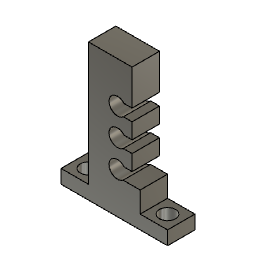
Horizantal Holder design v7 (Autodesk Fusion 360 archive; units mm, degrees)
design "Single Julia design"
Autodesk Fusion 360 part; units mm, degrees
box "BoxPrimitive2" add length 25.4 width 76.2 height 2.54 placed x (0, 0, 1) y (1, 0, 0) z (0, 1, 0) at (0, 0, 0)
sketch "Sketch3" plane through (0, 2.54, 0) normal (0, 1, 0) x (-1, 0, 0)
  line L0 (0, 25.4) -> (-76.2, 25.4)
  line L1 (-76.2, 0) -> (0, 0)
  line L2 (0, 0) -> (0, 25.4)
  line L3 (-29.21, 12.7) -> (-19.05, 12.7)
  line L4 (-19.05, 12.7) -> (-19.05, 25.4)
  line L5 (-19.05, 25.4) -> (-15.875, 25.4)
  line L6 (-15.875, 25.4) -> (-15.875, 0)
  line L7 (-15.875, 0) -> (-19.05, 0)
  line L8 (-19.05, 0) -> (-19.05, 12.7)
  line L9 (-15.875, 12.7) -> (-12.065, 12.7)
  line L10 (-12.065, 12.7) -> (-12.065, 25.4)
  line L11 (-12.065, 12.7) -> (-12.065, 0)
  line L12 (-17.4625, 25.4) -> (-17.4625, 0)
  circle A0 centre (-17.4625, 12.7) radius 1.5875
  circle A1 centre (-17.4625, 17.78) radius 1.5875
  circle A2 centre (-17.4625, 7.62) radius 1.5875
  line L13 (-19.05, 0) -> (-24.13, 0)
  line L14 (-24.13, 0) -> (-24.13, 2.54)
  line L15 (-24.13, 2.54) -> (-19.05, 2.54)
  line L16 (-19.05, 2.54) -> (-19.05, 0)
  line L17 (-19.05, 0) -> (-24.13, 0)
  line L18 (-24.13, 0) -> (-24.13, 2.54)
  dimension "d29" = 10.16
  dimension "d30" = 3.175
  dimension "d31" = 3.175
  dimension "d32" = 3.81
  dimension "d51" = 3.175
  dimension "d52" = 3.175
  dimension "d53" = 3.175
  dimension "d80" = 5.08
  dimension "d81" = 2.54
  constraint perpendicular L3 L4
  constraint perpendicular L4 L5
  constraint coincident L1 L6.end
  constraint perpendicular L1 L6
  constraint perpendicular L6 L7
  constraint midpoint L6 L9.start
  constraint perpendicular L6 L9
  constraint coincident L0 L10.end
  constraint perpendicular L0 L10
  constraint coincident L1 L11.end
  constraint perpendicular L1 L11
  constraint midpoint L5 L12.start
  constraint midpoint L7 L12.end
  constraint midpoint L12 A0.centre
  constraint coincident L12 A1.centre
  constraint coincident L12 A2.centre
  constraint perpendicular L8 L13
  constraint perpendicular L1 L14
  constraint horizontal L15
  constraint vertical L16
  constraint horizontal L17
  constraint vertical L18
  measures "d29" distance of L3.start L3.end
  measures "d30" distance of L4.end L5.end
  measures "d31" distance of L6.end L7.end
  measures "d32" distance of L9.start L9.end
  measures "d51" diameter of A0
  measures "d52" diameter of A1
  measures "d53" diameter of A2
  measures "d80" distance of L7.end L13.end
  measures "d81" distance of L13.end L14.end
scale "Scale1" factors (0.841667, 1, 1) about (0, 2.54, 25.4) bodies 1
move_body "Move1" bodies 1 to x (1, 0, 0) y (0, 1, 0) z (0, 0, 1) at (12.065, 0, 0)
extrude "Extrude1" cut sketch "Sketch3" against normal blind 12.7 contours L12 A1 | L12 A0 | L12 A1 | L12 A2 | L12 A0 | L12 A2
sketch "Sketch4" plane through (76.2, 0, 0) normal (1, 0, 0) x (0, 1, 0)
  line L0 (2.54, 25.4) -> (0, 25.4)
  line L1 (0, 25.4) -> (0, 0)
  line L2 (0, 0) -> (2.54, 0)
  line L3 (2.54, 0) -> (2.54, 25.4)
  line L4 (2.54, 0) -> (2.54, 2.54)
  line L5 (0, 2.54) -> (2.54, 2.54)
  line L6 (0, 2.54) -> (0, 0)
  line L7 (2.54, 0) -> (0, 0)
  dimension "d56" = 2.54
  constraint coincident L2.end L3.start
  constraint coincident L3 L4.end
  constraint coincident L1 L5.start
  constraint perpendicular L4 L5
  constraint coincident L1.end L2.start
  measures "d56" distance of L2.end L4.end
extrude "Extrude2" add sketch "Sketch4" along normal blind 5.08 contours L1 L2 L3 L4 L5 L6 L7
sketch "Sketch5" plane through (12.065, 0, 0) normal (-1, 0, 0) x (0, -1, 0)
  line L0 (-2.54, 0) -> (0, 0)
  line L1 (0, 0) -> (0, 25.4)
  line L2 (0, 25.4) -> (-2.54, 25.4)
  line L3 (-2.54, 25.4) -> (-2.54, 0)
  line L4 (0, 0) -> (0, 2.54)
  line L5 (0, 2.54) -> (-2.54, 2.54)
  line L6 (-2.54, 0) -> (-2.54, 2.54)
  line L7 (-2.54, 0) -> (0, 0)
  dimension "d59" = 2.54
  constraint coincident L0.end L1.start
  constraint perpendicular L0 L4
  constraint coincident L3 L5.end
  constraint perpendicular L3 L5
  constraint coincident L0.start L3.end
  measures "d59" distance of L0.end L4.end
extrude "Extrude3" add sketch "Sketch5" along normal blind 5.08 contours L0 L1 L3 L4 L5 L6 L7
move_face "MoveFace1" by (0, 2.54, 0) 1 faces at (57.15, 2.54, 13.5467)
sketch "Sketch7" plane through (0, 0, 2.54) normal (0, 0, 1) x (-1, 0, 0)
  line L0 (-76.2, -5.08) -> (-76.2, 0)
  line L1 (-76.2, 0) -> (-81.28, 0)
  line L2 (-81.28, 0) -> (-81.28, -5.08)
  line L3 (-81.28, -5.08) -> (-76.2, -5.08)
  line L4 (-81.28, -5.08) -> (-81.28, -2.54)
  line L5 (-78.74, -2.54) -> (-78.74, -5.08)
  circle A0 centre (-78.74, -2.54) radius 1.5
  dimension "d63" = 3
  constraint coincident L2.end L3.start
  constraint midpoint L2 L4.end
  constraint midpoint L3 L5.end
  constraint perpendicular L3 L5
  constraint coincident L5.start A0.centre
  measures "d63" diameter of A0
sketch "Sketch8" plane through (0, 0, 2.54) normal (0, 0, 1) x (-1, 0, 0)
  line L0 (-12.065, 0) -> (-12.065, -5.08)
  line L1 (-12.065, -5.08) -> (-6.985, -5.08)
  line L2 (-6.985, -5.08) -> (-6.985, 0)
  line L3 (-6.985, 0) -> (-12.065, 0)
  line L4 (-6.985, -2.54) -> (-9.525, -2.54)
  circle A0 centre (-9.525, -2.54) radius 1.5
  dimension "d64" = 3
  constraint midpoint L2 L4.start
  constraint perpendicular L2 L4
  constraint coincident L4.end A0.centre
  measures "d64" diameter of A0
extrude "Extrude4" cut sketch "Sketch8" sketch "Sketch7" against normal blind 5 contours A0 of sketch 2 contours A0
sketch "Sketch9" plane through (0, 0, 0) normal (0, 1, 0) x (1, 0, 0)
  line L0 (18.6768, -18.816) -> (20.1542, -18.816)
  line L1 (20.1542, -18.816) -> (20.1542, -26.2967)
  line L2 (20.1542, -26.2967) -> (21.6542, -26.2967)
  line L3 (21.6542, -26.2967) -> (21.6542, -16.6091)
  line L4 (18.1034, -16.6091) -> (18.1034, -18.816)
  line L5 (18.1034, -18.816) -> (18.6768, -18.816)
  line L6 (18.1034, -11.5091) -> (18.1034, -13.716)
  line L7 (18.1034, -13.716) -> (18.6768, -13.716)
  line L8 (18.6768, -13.716) -> (20.1542, -13.716)
  line L9 (20.1542, -13.716) -> (20.1542, -16.6091)
  line L10 (20.1542, -16.6091) -> (18.1034, -16.6091)
  line L11 (18.1034, -8.616) -> (18.6768, -8.616)
  line L12 (18.6768, -8.616) -> (20.1542, -8.616)
  line L13 (21.6542, -6.4091) -> (18.1034, -6.4091)
  line L14 (18.1034, -6.4091) -> (18.1034, -8.616)
  line L15 (21.6542, -6.4091) -> (21.6542, -16.6091)
  line L16 (20.1542, -8.616) -> (20.1542, -11.5091)
  line L17 (20.1542, -11.5091) -> (18.1034, -11.5091)
  dimension "d67" = 1.5
  constraint horizontal L0
  constraint perpendicular L0 L1
  constraint perpendicular L1 L2
  constraint perpendicular L2 L3
  constraint perpendicular L0 L4
  constraint perpendicular L4 L5
  constraint horizontal L8
  constraint perpendicular L6 L8
  constraint perpendicular L6 L7
  constraint perpendicular L8 L9
  constraint perpendicular L4 L10
  constraint horizontal L12
  constraint perpendicular L12 L14
  constraint perpendicular L11 L14
  constraint perpendicular L13 L15
  constraint perpendicular L12 L16
  constraint perpendicular L6 L17
  measures "d67" distance of L1.end L2.end
extrude "Extrude5" cut sketch "Sketch9" along normal blind 11
sketch "Sketch10" plane through (0, 0, 0) normal (0, -1, 0) x (1, 0, 0)
  line L0 (18.6823, 13.716) -> (20.1542, 13.716)
  line L1 (20.1542, 13.716) -> (20.1542, 16.6091)
  line L2 (20.1542, 16.6091) -> (18.5345, 16.6091)
  arc A0 (18.6654, 18.816) -> (18.5345, 16.6091) centre (17.4625, 17.78) ccw
  line L3 (18.6654, 18.816) -> (20.1542, 18.816)
  line L4 (20.1542, 18.816) -> (20.1542, 25.4)
  line L5 (20.1542, 25.4) -> (12.065, 25.4)
  line L6 (12.065, 25.4) -> (12.065, 2.54)
  line L7 (12.065, 2.54) -> (6.985, 2.54)
  line L8 (6.985, 2.54) -> (6.985, 0)
  line L9 (6.985, 0) -> (81.28, 0)
  line L10 (81.28, 0) -> (81.28, 2.54)
  line L11 (81.28, 2.54) -> (76.2, 2.54)
  line L12 (76.2, 2.54) -> (76.2, 25.4)
  line L13 (76.2, 25.4) -> (21.6542, 25.4)
  line L14 (21.6542, 25.4) -> (21.6542, 6.4091)
  line L15 (21.6542, 6.4091) -> (18.4891, 6.4091)
  arc A1 (18.6987, 8.616) -> (18.4891, 6.4091) centre (17.4625, 7.62) ccw
  line L16 (18.6987, 8.616) -> (20.1542, 8.616)
  line L17 (20.1542, 8.616) -> (20.1542, 11.5091)
  line L18 (20.1542, 11.5091) -> (18.5122, 11.5091)
  arc A2 (18.6823, 13.716) -> (18.5122, 11.5091) centre (17.4625, 12.7) ccw
  line L19 (21.6542, 25.4) -> (81.28, 25.4)
  line L20 (81.28, 25.4) -> (81.28, 0)
  line L21 (81.28, 0) -> (21.6542, 0)
  line L22 (21.6542, 0) -> (21.6542, 25.4)
  constraint horizontal L19
  constraint vertical L20
  constraint horizontal L21
  constraint vertical L22
  constraint coincident L9.end L10.start
  constraint coincident L13.end L14.start
extrude "Extrude6" cut sketch "Sketch10" against normal blind 7 contours L9 L10 L11 L12 L13 L14 L19 L20 L21 L22
sketch "Sketch11" plane through (0, 0, 0) normal (0, -1, 0) x (1, 0, 0)
  line L0 (21.6542, 0) -> (21.6542, 6.4091)
  line L1 (21.6542, 6.4091) -> (18.4891, 6.4091)
  arc A0 (18.6987, 8.616) -> (18.4891, 6.4091) centre (17.4625, 7.62) ccw
  line L2 (18.6987, 8.616) -> (20.1542, 8.616)
  line L3 (20.1542, 8.616) -> (20.1542, 11.5091)
  line L4 (20.1542, 11.5091) -> (18.5122, 11.5091)
  arc A1 (18.6823, 13.716) -> (18.5122, 11.5091) centre (17.4625, 12.7) ccw
  line L5 (18.6823, 13.716) -> (20.1542, 13.716)
  line L6 (20.1542, 13.716) -> (20.1542, 16.6091)
  line L7 (20.1542, 16.6091) -> (18.5345, 16.6091)
  arc A2 (18.6654, 18.816) -> (18.5345, 16.6091) centre (17.4625, 17.78) ccw
  line L8 (18.6654, 18.816) -> (20.1542, 18.816)
  line L9 (20.1542, 18.816) -> (20.1542, 25.4)
  line L10 (20.1542, 25.4) -> (12.065, 25.4)
  line L11 (12.065, 25.4) -> (12.065, 2.54)
  line L12 (12.065, 2.54) -> (6.985, 2.54)
  line L13 (6.985, 2.54) -> (6.985, 0)
  line L14 (6.985, 0) -> (21.6542, 0)
  line L15 (6.985, 2.54) -> (30, 2.54)
  line L16 (21.6542, 2.54) -> (26.7342, 2.54)
  line L17 (26.7342, 2.54) -> (26.7342, 0)
  line L18 (26.7342, 0) -> (21.6542, 0)
  line L19 (21.6542, 0) -> (21.6542, 2.54)
  dimension "d84" = 5.08
  constraint coincident L12.end L13.start
  constraint perpendicular L0 L15
  constraint horizontal L16
  constraint vertical L17
  constraint horizontal L18
  constraint vertical L19
  constraint coincident L15 L16.start
  constraint coincident L0 L16.start
  measures "d84" distance of L16.start L16.end
extrude "Extrude7" add sketch "Sketch11" against normal blind 5.08 contours L0 L15 L16 L17 L18 L19
sketch "Sketch12" plane through (0, 0, 2.54) normal (0, 0, 1) x (-1, 0, 0)
  line L0 (-21.6542, 0) -> (-26.7342, 0)
  line L1 (-26.7342, 0) -> (-26.7342, -5.08)
  line L2 (-26.7342, -5.08) -> (-21.6542, -5.08)
  line L3 (-21.6542, -5.08) -> (-21.6542, 0)
  line L4 (-26.7342, -2.54) -> (-24.1942, -2.54)
  circle A0 centre (-24.1942, -2.54) radius 1.5
  dimension "d87" = 2.54
  dimension "d88" = 3
  constraint midpoint L1 L4.start
  constraint perpendicular L1 L4
  constraint coincident L4.end A0.centre
  measures "d87" distance of L4.start L4.end
  measures "d88" diameter of A0
extrude "Extrude8" cut sketch "Sketch12" against normal blind 4 contours A0
sketch "Sketch13" plane through (0, 0, 0) normal (0, 0, -1) x (1, 0, 0)
  circle A0 centre (24.1942, -2.54) radius 1.5
  line L0 (26.7342, 0) -> (6.985, 0)
  line L1 (6.985, 0) -> (6.985, -5.08)
  line L2 (6.985, -5.08) -> (26.7342, -5.08)
  line L3 (26.7342, -5.08) -> (26.7342, 0)
  circle A1 centre (9.525, -2.54) radius 1.5

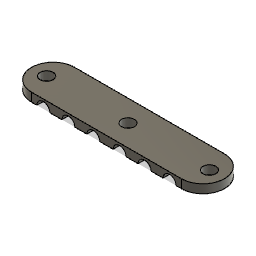
design "ESc indie mount"
Autodesk Fusion 360 part; units mm, degrees
sketch "Sketch1" plane through (0, 0, 0) normal (0, 0, 1) x (1, 0, 0)
  line L0 (0, 0) -> (17.1, 0)
  line L1 (17.1, 0) -> (17.1, 2)
  line L2 (17.1, 2) -> (0, 2)
  line L3 (0, 2) -> (0, 0)
  line L4 (0, 0) -> (1.25, 0)
  line L5 (1.25, 0) -> (2.75, 0)
  circle A0 centre (2.75, 0) radius 1.5
  line L6 (4.25, 0) -> (7.05, 0)
  line L7 (7.05, 0) -> (8.55, 0)
  circle A1 centre (8.55, 0) radius 1.5
  line L8 (10.05, 0) -> (12.85, 0)
  line L9 (12.85, 0) -> (14.35, 0)
  circle A2 centre (14.35, 0) radius 1.5
  line L10 (15.85, 0) -> (17.1, 0)
  line L11 (15.85, 0) -> (17.4, 0)
  line L12 (17.4, 0) -> (18.95, 0)
  line L13 (18.95, 0) -> (17.1, 0)
  line L14 (17.1, 0) -> (17.1, 2)
  line L15 (17.1, 2) -> (18.95, 2)
  line L16 (18.95, 2) -> (18.95, 0)
  line L17 (17.1, 2) -> (34.2, 2)
  line L18 (34.2, 0) -> (17.1, 0)
  line L19 (18.95, 0) -> (20.45, 0)
  circle A3 centre (20.45, 0) radius 1.5
  line L20 (21.95, 0) -> (24.75, 0)
  line L21 (24.75, 0) -> (26.25, 0)
  circle A4 centre (26.25, 0) radius 1.5
  line L22 (27.75, 0) -> (30.55, 0)
  line L23 (30.55, 0) -> (32.05, 0)
  circle A5 centre (32.05, 0) radius 1.5
  line L24 (33.55, 0) -> (34.8, 0)
  line L25 (34.8, 0) -> (33.05, 0)
  line L26 (33.05, 0) -> (33.05, 2)
  line L27 (33.05, 2) -> (34.8, 2)
  line L28 (34.8, 2) -> (34.8, 0)
  dimension "d1" = 17.1
  dimension "d2" = 2
  dimension "d3" = 1.25
  dimension "d4" = 1.5
  dimension "d5" = 2.8
  dimension "d6" = 1.5
  dimension "d7" = 2.8
  dimension "d8" = 1.5
  dimension "d32" = 1.55
  dimension "d33" = 1.55
  dimension "d39" = 1.5
  dimension "d41" = 2.8
  dimension "d42" = 1.5
  dimension "d43" = 2.8
  dimension "d44" = 1.5
  dimension "d45" = 1.25
  constraint horizontal L0
  constraint vertical L1
  constraint horizontal L2
  constraint vertical L3
  constraint coincident L0.start L3.end
  constraint perpendicular L3 L4
  constraint parallel L0 L5
  constraint coincident L5.end A0.centre
  constraint coincident L4.end A0
  constraint coincident L0 L6.start
  constraint coincident A0 L6.start
  constraint parallel L0 L6
  constraint parallel L0 L7
  constraint coincident L7.end A1.centre
  constraint coincident L6.end A1
  constraint coincident A1 L8.start
  constraint coincident L0 L8.start
  constraint parallel L0 L8
  constraint parallel L0 L9
  constraint coincident L9.end A2.centre
  constraint coincident L8.end A2
  constraint coincident L0 L10.start
  constraint coincident A2 L10.start
  constraint perpendicular L1 L11
  constraint perpendicular L1 L12
  constraint horizontal L13
  constraint vertical L14
  constraint horizontal L15
  constraint vertical L16
  constraint symmetric L0.start L14 L18.start
  constraint symmetric L0.end L14 L1.start
  constraint symmetric L1.end L14 L2.start
  constraint symmetric L2.end L14 L17.end
  constraint perpendicular L16 L19
  constraint coincident L19.end A3.centre
  constraint coincident L12.end A3
  constraint coincident L18 L20.start
  constraint coincident A3 L20.start
  constraint parallel L18 L20
  constraint parallel L18 L21
  constraint coincident L21.end A4.centre
  constraint coincident L20.end A4
  constraint coincident A4 L22.start
  constraint coincident L18 L22.start
  constraint parallel L18 L22
  constraint parallel L18 L23
  constraint coincident L23.end A5.centre
  constraint coincident L22.end A5
  constraint coincident A5 L24.start
  constraint coincident L18 L24.start
  constraint horizontal L25
  constraint vertical L26
  constraint horizontal L27
  constraint vertical L28
  constraint coincident L17 L26.end
  measures "d1" distance of L0.start L0.end
  measures "d2" distance of L0.start L2.end
  measures "d3" distance of L0.start L4.end
  measures "d4" distance of L4.end L5.end
  measures "d5" distance of L6.start L6.end
  measures "d6" distance of L6.end L7.end
  measures "d7" distance of L8.start L8.end
  measures "d8" distance of L8.end L9.end
  measures "d32" distance of L10.start L11.end
  measures "d33" distance of L11.end L12.end
  measures "d39" distance of L12.end L19.end
  measures "d41" distance of L20.start L20.end
  measures "d42" distance of L20.end L21.end
  measures "d43" distance of L22.start L22.end
  measures "d44" distance of L22.end L23.end
  measures "d45" distance of L24.start L24.end
extrude "Extrude1" add sketch "Sketch1" along normal blind 10 contours L0 L1 L2 L3 L4 A0 L6 A1 L8 A2 L10 L11 L14 | L1 L11 L12 L13 L14 L15 L16 L17 L18 | L16 L17 L18 A3 L20 A4 L22 A5 L26 | L17 L18 A5 L24 L25 L26 L27 L28
sketch "Sketch10" plane through (0, 0, 0) normal (0, -1, 0) x (1, 0, 0)
  line L0 (15.85, 0) -> (18.95, 0)
  line L1 (18.95, 0) -> (18.95, 10)
  line L2 (18.95, 10) -> (15.85, 10)
  line L3 (15.85, 10) -> (15.85, 0)
  line L4 (15.85, 0) -> (18.95, 0)
  line L5 (17.4, 0) -> (17.4, 10)
  circle A0 centre (17.4, 5) radius 1.5
  dimension "d46" = 3
  constraint coincident L0.start L3.end
  constraint coincident L0.end L1.start
  constraint midpoint L0 L5.start
  constraint midpoint L2 L5.end
  constraint midpoint L5 A0.centre
  measures "d46" diameter of A0
extrude "Extrude6" cut sketch "Sketch10" against normal blind 2.6 contours L5 A0 | L5 A0
sketch "Sketch7" plane through (0, 2, 0) normal (0, 1, 0) x (-1, 0, 0)
  line L0 (-34.8, 0) -> (0, 0)
  line L1 (0, 0) -> (0, 10)
  line L2 (0, 10) -> (-34.8, 10)
  line L3 (0, 0) -> (0, 10)
  line L4 (0, 0) -> (-34.8, 0)
  line L5 (-17.4, 0) -> (-17.4, 10)
  circle A0 centre (0, 5) radius 5
  line L6 (0, 5) -> (5, 5)
  circle A1 centre (-17.4, 5) radius 1.5
  line L7 (-34.8, 10) -> (-34.8, 0)
  line L8 (2.5, 5) -> (0, 5)
  line L9 (2.5, 5) -> (2.1, 5)
  line L10 (2.5, 5) -> (0.5, 5)
  line L11 (2.5, 5) -> (1, 5)
  line L12 (1, 5) -> (1.5, 5)
  circle A2 centre (1.5, 5) radius 1.5
  circle A3 centre (-34.8, 5) radius 5
  circle A4 centre (-36.3, 5) radius 1.5
  line L13 (0, 10) -> (-1.25, 10)
  line L14 (-1.25, 10) -> (-1.25, 0)
  line L15 (5, 5) -> (-1.25, 5)
  dimension "d49" = 0.4
  dimension "d50" = 2
  dimension "d52" = 0.5
  constraint coincident L0.end L1.start
  constraint coincident L1.end L2.start
  constraint coincident L0.start L4.end
  constraint midpoint L4 L5.start
  constraint midpoint L2 L5.end
  constraint midpoint L3 A0.centre
  constraint coincident L1.end A0
  constraint coincident A0.centre L6.start
  constraint coincident A0 L6.end
  constraint perpendicular L3 L6
  constraint parallel L8 L9
  constraint parallel L8 L10
  constraint coincident L6 L11.end
  constraint parallel L8 L12
  constraint coincident L12.end A2.centre
  constraint coincident A0.centre A2
  constraint symmetric L5 A0 A3
  constraint symmetric L5 A2 A4
  constraint coincident L2 L13.end
  constraint tangent A0 L13
  constraint coincident L4 L14.end
  constraint perpendicular L4 L14
  constraint midpoint L14 L15.end
  constraint perpendicular L14 L15
  measures "d49" distance of L8.start L9.end
  measures "d50" distance of L8.start L10.end
  measures "d52" distance of L11.end L12.end
extrude "Extrude5" add sketch "Sketch7" against normal blind 2 contours L7 A3 | L1 L3 A0 L6 A2 L15 | L1 L3 A0 L6 A2 L15 picked at (-35.3657, 1.2198)
